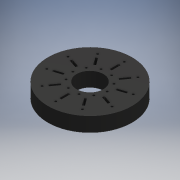
# Autodesk Inventor part: SG03
Saved by Autodesk Inventor 2017 (Build 210142000, 142)
## iProperties
Created: 2019-10-04
Part Number: SG03
Material: Rubber
Document SubType Name: Modeling
Designer: Dell
Density: 0.93 g/cm^3
Appearance: Rubber - Black
Author: Dell
Autodesk Inventor part; units mm, degrees
ref_plane "YZ Plane" through (0, 0, 0) normal (1, 0, 0) x (0, 1, 0)
ref_plane "XZ Plane" through (0, 0, 0) normal (0, 1, 0) x (-1, 0, 0)
ref_plane "XY Plane" through (0, 0, 0) normal (0, 0, 1) x (1, 0, 0)
sketch "Sketch1" plane through (0, 0, 0) normal (0, 0, 1) x (1, 0, 0)
  circle A0 centre (0, 0) radius 11.75
  circle A1 centre (0, 0) radius 36.75
  dimension "d0" = 23.5
  dimension "d1" = 73.5
  constraints: 2 centre point, 2 coincident
  measures "d0" diameter of A0
  measures "d1" diameter of A1
extrude "Extrusion1" add sketch "Sketch1" along normal blind 12.7
sketch "Sketch2" plane through (0, 0, 12.7) normal (0, 0, 1) x (1, 0, 0)
  circle A0 centre (15, 0) radius 1
  circle A1 centre (0, 30) radius 1
  circle A2 centre (12.1353, 8.8168) radius 1
  circle A3 centre (4.6353, 14.2658) radius 1
  circle A4 centre (-4.6353, 14.2658) radius 1
  circle A5 centre (-12.1353, 8.8168) radius 1
  circle A6 centre (-15, 0) radius 1
  circle A7 centre (-12.1353, -8.8168) radius 1
  circle A8 centre (-4.6353, -14.2658) radius 1
  circle A9 centre (4.6353, -14.2658) radius 1
  circle A10 centre (12.1353, -8.8168) radius 1
  circle A11 centre (-17.6336, 24.2705) radius 1
  circle A12 centre (-28.5317, 9.2705) radius 1
  circle A13 centre (-28.5317, -9.2705) radius 1
  circle A14 centre (-17.6336, -24.2705) radius 1
  circle A15 centre (0, -30) radius 1
  circle A16 centre (17.6336, -24.2705) radius 1
  circle A17 centre (28.5317, -9.2705) radius 1
  circle A18 centre (28.5317, 9.2705) radius 1
  circle A19 centre (17.6336, 24.2705) radius 1
  point P0 (0, 0)
  dimension "d4" = 2
  dimension "d5" = 2
  dimension "d6" = 15
  dimension "d7" = 30
  dimension "d10" = 360
  dimension "d14" = 360
  constraints: 20 centre point, 1 horizontal alignment, 1 vertical alignment, 42 other
  measures "d4" diameter of A0
  measures "d5" diameter of A1
  measures "d6" distance of point (0, 0) A0.centre
  measures "d7" distance of A1.centre point (0, 0)
extrude "Extrusion2" cut sketch "Sketch2" against normal through all
sketch "Sketch3" plane through (0, 0, 12.7) normal (0, 0, 1) x (1, 0, 0)
  line L0 (-1, 18) -> (1, 18)
  line L1 (1, 18) -> (1, 26)
  line L2 (1, 26) -> (-1, 26)
  line L3 (-1, 26) -> (-1, 18)
  line L4 (-11.3892, 13.9745) -> (-9.7711, 15.1501)
  line L5 (-9.7711, 15.1501) -> (-14.4734, 21.6222)
  line L6 (-14.4734, 21.6222) -> (-16.0914, 20.4467)
  line L7 (-16.0914, 20.4467) -> (-11.3892, 13.9745)
  line L8 (-17.428, 4.6112) -> (-16.81, 6.5134)
  line L9 (-16.81, 6.5134) -> (-24.4185, 8.9855)
  line L10 (-24.4185, 8.9855) -> (-25.0365, 7.0834)
  line L11 (-25.0365, 7.0834) -> (-17.428, 4.6112)
  line L12 (-16.81, -6.5134) -> (-17.428, -4.6112)
  line L13 (-17.428, -4.6112) -> (-25.0365, -7.0834)
  line L14 (-25.0365, -7.0834) -> (-24.4185, -8.9855)
  line L15 (-24.4185, -8.9855) -> (-16.81, -6.5134)
  line L16 (-9.7711, -15.1501) -> (-11.3892, -13.9745)
  line L17 (-11.3892, -13.9745) -> (-16.0914, -20.4467)
  line L18 (-16.0914, -20.4467) -> (-14.4734, -21.6222)
  line L19 (-14.4734, -21.6222) -> (-9.7711, -15.1501)
  line L20 (1, -18) -> (-1, -18)
  line L21 (-1, -18) -> (-1, -26)
  line L22 (-1, -26) -> (1, -26)
  line L23 (1, -26) -> (1, -18)
  line L24 (11.3892, -13.9745) -> (9.7711, -15.1501)
  line L25 (9.7711, -15.1501) -> (14.4734, -21.6222)
  line L26 (14.4734, -21.6222) -> (16.0914, -20.4467)
  line L27 (16.0914, -20.4467) -> (11.3892, -13.9745)
  line L28 (17.428, -4.6112) -> (16.81, -6.5134)
  line L29 (16.81, -6.5134) -> (24.4185, -8.9855)
  line L30 (24.4185, -8.9855) -> (25.0365, -7.0834)
  line L31 (25.0365, -7.0834) -> (17.428, -4.6112)
  line L32 (16.81, 6.5134) -> (17.428, 4.6112)
  line L33 (17.428, 4.6112) -> (25.0365, 7.0834)
  line L34 (25.0365, 7.0834) -> (24.4185, 8.9855)
  line L35 (24.4185, 8.9855) -> (16.81, 6.5134)
  line L36 (9.7711, 15.1501) -> (11.3892, 13.9745)
  line L37 (11.3892, 13.9745) -> (16.0914, 20.4467)
  line L38 (16.0914, 20.4467) -> (14.4734, 21.6222)
  line L39 (14.4734, 21.6222) -> (9.7711, 15.1501)
  point P0 (0, 0)
  point P1 (0, 18)
  point P2 (-10.5801, 14.5623)
  point P3 (-17.119, 5.5623)
  point P4 (-17.119, -5.5623)
  point P5 (-10.5801, -14.5623)
  point P6 (0, -18)
  point P7 (10.5801, -14.5623)
  point P8 (17.119, -5.5623)
  point P9 (17.119, 5.5623)
  point P10 (10.5801, 14.5623)
  dimension "d18" = 18
  dimension "d19" = 26
  dimension "d20" = 2
  dimension "d23" = 360
  constraints: 80 end point, 3 perpendicular, 1 horizontal, 1 midpoint, 1 vertical alignment, 91 other
  measures "d18" distance from line of point (0, 0) L0
  measures "d19" distance from line of point (0, 0) L2
  measures "d20" distance of L0.start L0.end
extrude "Extrusion3" cut sketch "Sketch3" against normal through all
body "Solid1"
